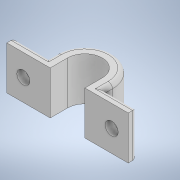
# Autodesk Inventor part: Part_B5
Saved by Autodesk Inventor 2022.6 (Build 266554010, 554A)
## iProperties
Created: 2025-05-30
Part Number: Part_B5
Material: Generic
Document SubType Name: Modeling
Designer: khinm
Density: 1 g/cm^3
Appearance: Default
Author: khinm
Autodesk Inventor part; units mm, degrees
ref_plane "YZ Plane" through (0, 0, 0) normal (1, 0, 0) x (0, 1, 0)
ref_plane "XZ Plane" through (0, 0, 0) normal (0, 1, 0) x (-1, 0, 0)
ref_plane "XY Plane" through (0, 0, 0) normal (0, 0, 1) x (1, 0, 0)
sketch "Sketch1" plane through (0, 0, 0) normal (0, 1, 0) x (-1, 0, 0)
  arc A0 (-4, 0) -> (4, 0) centre (0, 0) ccw
  line L0 (-4, 4) -> (-14, 4)
  line L1 (4, 4) -> (14, 4)
  line L2 (14, 2) -> (6.3562, 2)
  line L3 (-6.3562, 2) -> (-14, 2)
  line L4 (4, 0) -> (4, 4)
  line L5 (-4, 0) -> (-4, 4)
  line L6 (6.3562, 0) -> (6.3562, 2)
  line L7 (-6.3562, 0) -> (-6.3562, 2)
  arc A1 (-6.3562, 0) -> (6.3562, 0) centre (0, 0) ccw
  line L8 (14, 2) -> (14, 4)
  line L9 (-14, 2) -> (-14, 4)
  dimension "d0" = 8
  dimension "d2" = 2
  dimension "d3" = 10
  dimension "d4" = 10
  dimension "d5" = 6.3562
  dimension "d6" = 2
  constraints: 20 end point, 6 perpendicular, 6 tangent, 4 point on circle, 2 centre point, 2 coincident, 2 horizontal
  measures "d0" diameter of A0
  measures "d2" distance between parallel lines of L1 L2
  measures "d3" distance of L0.start L0.end
  measures "d4" distance of L1.start L1.end
  measures "d5" radius of A1
  measures "d6" distance between parallel lines of L0 L3
extrude "Extrusion1" add sketch "Sketch1" along normal mid plane 10
sketch "Sketch2" plane through (14, 5, 2) normal (0, 0, -1) x (-1, 0, 0)
  line L0 (0, -10) -> (0, 0) projected
  line L1 (0, 0) -> (7.6438, 0) projected
  point P0 (14, -5)
  point P1 (3.8219, -5)
  point P2 (0, -5)
  point P3 (3.8219, 0)
  constraints: 2 midpoint, 1 horizontal alignment, 1 vertical alignment
hole "Hole1" at (10.1781, 0, 2) direction (0, 0, 1) diameter 3 depth 2
mirror "Mirror1" about plane through (0, 0, 0) normal (1, 0, 0) of "Hole1"
fillet "Fillet1" radius 1 12 edges at (10.1781, 5, 2) (14, 0, 2) (10.1781, -5, 2) (-10.1781, 5, 2) (-14, 0, 2) (-10.1781, -5, 2) (-6.3562, 5, 1) (6.3562, 5, 1) (0, 5, -6.3562) (6.3562, -5, 1) (-6.3562, -5, 1) (0, -5, -6.3562)
body "Solid1"
